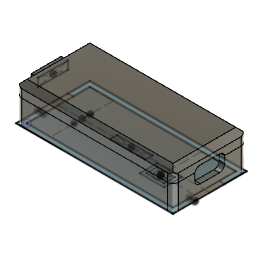
sim_case v2 (Autodesk Fusion 360 design; units mm, degrees)
Autodesk Fusion 360 part; units mm, degrees
sketch "Sketch1" plane through (0, 0, 0) normal (0, 0, 1) x (1, 0, 0)
  line L0 (0, 0) -> (53.5, 0)
  line L1 (53.5, 0) -> (53.5, 23)
  line L2 (53.5, 23) -> (0, 23)
  line L3 (0, 23) -> (0, 0)
  line L4 (-2, -2) -> (55.5, -2)
  line L5 (55.5, -2) -> (55.5, 25)
  line L6 (55.5, 25) -> (-2, 25)
  line L7 (-2, 25) -> (-2, -2)
  line L8 (55.5, 11.5) -> (-2, 11.5) construction
  line L9 (55.5, 11.5) -> (55.5, 17) construction
  line L10 (55.5, 17) -> (53.5, 17)
  line L11 (-2, 11.5) -> (-2, 17) construction
  line L12 (-2, 17) -> (0, 17)
  line L13 (-2, 6) -> (0, 6)
  line L14 (55.5, 6) -> (53.5, 6)
  line L15 (53.5, 23) -> (41, 23) construction
  line L16 (41, 23) -> (41, 8) construction
  line L17 (41, 8) -> (53.5, 8) construction
  line L18 (53.5, 8) -> (53.5, 23) construction
  line L19 (0, 23) -> (8.7, 23) construction
  line L20 (8.7, 23) -> (8.7, 0) construction
  line L21 (8.7, 11.5) -> (8.7, 14.5) construction
  circle A0 centre (8.7, 14.5) radius 0.5
  circle A1 centre (8.7, 8.5) radius 0.5
  circle A2 centre (41, 8) radius 2
  line L22 (33.25, 12.75) -> (20.25, 12.75)
  line L23 (20.25, 12.75) -> (20.25, 10.25)
  line L24 (20.25, 10.25) -> (33.25, 10.25)
  line L25 (33.25, 10.25) -> (33.25, 12.75)
  line L26 (33.25, 12.75) -> (20.25, 10.25) construction
  line L27 (20.25, 12.75) -> (33.25, 10.25) construction
  line L28 (-1, -1) -> (54.5, -1)
  line L29 (54.5, 24) -> (-1, 24)
  line L30 (-1, 17) -> (-1, 6) construction
  line L31 (54.5, -1) -> (54.5, 6)
  line L32 (54.5, 11.5) -> (54.5, 17) construction
  line L33 (54.5, 6) -> (54.5, 11.5) construction
  line L34 (-1, 6) -> (-1, -1)
  line L35 (-1, 24) -> (-1, 17)
  line L36 (54.5, 17) -> (54.5, 24)
  point P0 (41, 8)
  point P1 (8.7, 11.5)
  point P2 (26.75, 11.5)
  dimension "d1" = 53.5
  dimension "d2" = 23
  dimension "d3" = 2
  dimension "d4" = 5.5
  dimension "d5" = 5.5
  dimension "d6" = 12.5
  dimension "d7" = 15
  dimension "d10" = 8.7
  dimension "d11" = 3
  dimension "d12" = 1
  dimension "d13" = 4
  dimension "d14" = 13
  dimension "d15" = 2.5
  constraint horizontal L0
  constraint vertical L1
  constraint horizontal L2
  constraint vertical L3
  constraint coincident L0.start L3.end
  constraint midpoint L5 L8.start
  constraint midpoint L7 L8.end
  constraint perpendicular L8 L9
  constraint coincident L1 L10.end
  constraint perpendicular L1 L10
  constraint perpendicular L8 L11
  constraint coincident L3 L12.end
  constraint perpendicular L3 L12
  constraint symmetric L8 L9.end L14.start
  constraint symmetric L8 L10.end L14.end
  constraint symmetric L8 L11.end L13.start
  constraint symmetric L8 L12.end L13.end
  constraint horizontal L15
  constraint vertical L16
  constraint horizontal L17
  constraint vertical L18
  constraint coincident P0 L16.end
  constraint perpendicular L3 L19
  constraint coincident L0 L20.end
  constraint perpendicular L0 L20
  constraint midpoint L20 P1
  constraint coincident P1 L21.start
  constraint perpendicular L8 L21
  constraint coincident L21.end A0.centre
  constraint symmetric L8 A0 A1
  constraint horizontal L22
  constraint perpendicular L22 L23
  constraint parallel L22 L24
  constraint parallel L23 L25
  constraint coincident L26 P2
  constraint coincident L27 P2
  constraint midpoint L8 P2
  constraint parallel L0 L28
  constraint parallel L1 L31
  constraint parallel L2 L29
  constraint parallel L3 L30
  constraint coincident L14 L31.end
  constraint coincident L8 L32.start
  constraint coincident L13 L30.end
  constraint parallel L3 L34
  constraint coincident L12 L30.start
  constraint parallel L3 L35
  constraint coincident L10 L32.end
  measures "d1" distance of L0.start L0.end
  measures "d2" distance of L0.start L2.end
  measures "d4" distance of L8.start L9.end
  measures "d5" distance of L8.end L11.end
  measures "d6" distance of L1.end L15.end
  measures "d7" distance of L1.end L17.end
  measures "d10" distance of L2.end L19.end
  measures "d11" distance of P1 L21.end
  measures "d12" diameter of A0
  measures "d13" diameter of A2
  measures "d14" distance of L23.end L24.end
  measures "d15" distance of L22.end L23.end
extrude "Extrude1" add sketch "Sketch1" against normal blind 2 makes body 1
extrude "Extrude2" add sketch "Sketch1" along normal blind 9 contours L0 L1 L3 L13 L14 L28 L31 L34 | L1 L2 L3 L10 L12 L29 L35 L36 | L4 L5 L7 L13 L14 L28 L31 L34 | L5 L6 L7 L10 L12 L29 L35 L36 bodies 1
extrude "Extrude3" add sketch "Sketch1" along normal blind 6 contours L3 L7 L12 L13 bodies 1
extrude "Extrude4" add sketch "Sketch1" along normal blind 4.5 contours L1 L5 L10 L14 bodies 1
extrude "Extrude5" add sketch "Sketch1" along normal blind 2 from surface at 12 separate body contours L0 L1 L2 L3 | L0 L1 L3 L13 L14 L28 L31 L34 | L3 L7 L12 L13 | L1 L5 L10 L14 | L1 L2 L3 L10 L12 L29 L35 L36 | L4 L5 L7 L13 L14 L28 L31 L34 | L5 L6 L7 L10 L12 L29 L35 L36 | A0 | A1 | A2 | L22 L23 L24 L25 makes body 2
copy_body "Body->Comp1" bodies 1 removing the originals makes body 3 in component "Cover_top"
copy_body "Body->Comp2" bodies 2 removing the originals makes body 4 in component "Cover_bottom"
extrude "Extrude6" add sketch "Sketch1" along normal up to surface (3 mm away) from surface at 9 separate body contours L0 L1 L3 L13 L14 L28 L31 L34 | L1 L2 L3 L10 L12 L29 L35 L36 | L4 L5 L7 L13 L14 L28 L31 L34 | L5 L6 L7 L10 L12 L29 L35 L36 makes body 5 at (17.1667, -2, 10) makes body 6 at (36.3333, 25, 10)
extrude "Extrude7" add sketch "Sketch1" against normal blind 1.5 from surface at 12 contours L1 L5 L10 L14 bodies 6 5
combine "Combine1" operation add target body 4 tool bodies 6 in component "Cover_bottom"
extrude "Extrude1'" add sketch "Sketch1" against normal blind 3 from surface at 12 contours L3 L7 L12 L13 bodies 4 in component "Cover_bottom"
fillet "Fillet1" radius 2 2 edges at (54.5, 17, 4.5) (54.5, 6, 4.5) on bodies 3 in component "Cover_top"
fillet "Fillet1'" radius 2 2 edges at (54.5, 17, 10.5) (54.5, 6, 10.5) on bodies 4 in component "Cover_bottom"
chamfer "Chamfer1" distance 2 angle 45 4 edges at (26.75, -2, -2) (-2, 11.5, -2) (55.5, 11.5, -2) (26.75, 25, -2) on bodies 3 in component "Cover_top"
chamfer "Chamfer1'" distance 2 angle 45 4 edges at (26.75, -2, 14) (-2, 11.5, 14) (26.75, 25, 14) (55.5, 11.5, 14) on bodies 4 in component "Cover_bottom"
fillet "Fillet2" radius 2 4 edges at (-2, -2, 4.5) (-2, 25, 4.5) (55.5, 25, 4.5) (55.5, -2, 4.5) on bodies 3 in component "Cover_top"
fillet "Fillet2'" radius 2 4 edges at (-2, -2, 10.5) (-2, 25, 10.5) (55.5, 25, 10.5) (55.5, -2, 10.5) on bodies 4 in component "Cover_bottom"
extrude "Extrude1''" add sketch "Sketch1" along normal blind 1 from surface at 9 separate body contours L0 L1 L3 L13 L14 L28 L31 L34 | L1 L2 L3 L10 L12 L29 L35 L36 makes body 7 at (17.8333, 23.6667, 9) makes body 8 at (17.8333, -0.6667, 9) in component "Cover_top"
combine "Combine2" operation cut target body 4 tool bodies 7 8 keep tools in component "Cover_bottom"
combine "Combine1'" operation add target body 3 tool bodies 7 8 in component "Cover_top"
fillet "Fillet3" radius 1 4 edges at (-1, 24, 9.5) (54.5, 24, 9.5) (54.5, -1, 9.5) (-1, -1, 9.5) on bodies 3 in component "Cover_top"
sketch "Sketch2" plane through (0, 0, 0) normal (0, 0, 1) x (-1, 0, 0)
  line L0 (-53.5, 0) -> (-53.5, -23)
  line L1 (-53.5, -23) -> (0, -23)
  line L2 (0, -23) -> (0, 0)
  line L3 (0, 0) -> (-53.5, 0)
  circle A0 centre (-8.7, -14.5) radius 0.5
  circle A1 centre (-8.7, -8.5) radius 0.5
  line L4 (-33.25, -12.75) -> (-33.25, -10.25)
  line L5 (-33.25, -10.25) -> (-20.25, -10.25)
  line L6 (-20.25, -10.25) -> (-20.25, -12.75)
  line L7 (-20.25, -12.75) -> (-33.25, -12.75)
  circle A2 centre (-41, -8) radius 2
  line L8 (-44.25, -10) -> (-37.75, -10)
  line L9 (-37.75, -10) -> (-37.75, -6)
  line L10 (-37.75, -6) -> (-44.25, -6)
  line L11 (-44.25, -6) -> (-44.25, -10)
  line L12 (-44.25, -10) -> (-37.75, -6) construction
  line L13 (-37.75, -10) -> (-44.25, -6) construction
  line L14 (-36.55, -4.8) -> (-45.45, -4.8)
  line L15 (-45.45, -4.8) -> (-45.45, -11.2)
  line L16 (-45.45, -11.2) -> (-36.55, -11.2)
  line L17 (-36.55, -11.2) -> (-36.55, -4.8)
  point P0 (-41, -8)
  dimension "d49" = 6.5
  dimension "d50" = 4
  dimension "d51" = 1.2
  constraint horizontal L8
  constraint perpendicular L8 L9
  constraint parallel L8 L10
  constraint parallel L9 L11
  constraint coincident L12 P0
  constraint coincident L13 P0
  constraint coincident P0 A2.centre
  measures "d49" distance of L9.end L10.end
  measures "d50" distance of L8.end L9.end
extrude "Extrude1'''" add sketch "Sketch2" along normal blind 4.5 and the other way blind 3 separate body contours A2 makes body 9 in component "Button"
extrude "Extrude2'" add sketch "Sketch2" against normal blind 2 from surface at 4.5 contours A2 L8 L9 L10 | A2 L8 L10 L11 | L14 L15 L16 L17 bodies 9 in component "Button"
extrude "Extrude3'" add sketch "Sketch2" along normal blind 4 from surface at 4.5 contours L14 L15 L16 L17 bodies 9 in component "Button"
move_face "OffsetFaces1" offset -0.2 1 faces at (39.0025, 8.0997, 0.6667) on bodies 9 in component "Button"
sketch "Sketch3" plane through (-2, 0, 0) normal (-1, 0, 0) x (0, -1, 0)
  line L0 (-23, 12) -> (-23, 9)
  line L1 (-23, 9) -> (0, 9)
  line L2 (0, 9) -> (0, 12)
  line L3 (0, 12) -> (-23, 12)
  line L4 (-6, 10.5) -> (-17, 10.5)
  line L5 (-17, 10.5) -> (-17, 7.5)
  line L6 (-17, 7.5) -> (-6, 7.5)
  line L7 (-6, 7.5) -> (-6, 10.5)
  line L8 (-6, 10.5) -> (-17, 7.5) construction
  line L9 (-17, 10.5) -> (-6, 7.5) construction
  point P0 (-11.5, 9)
  dimension "d63" = 11
  dimension "d64" = 3
  constraint horizontal L4
  constraint perpendicular L4 L5
  constraint parallel L4 L6
  constraint parallel L5 L7
  constraint coincident L8 P0
  constraint coincident L9 P0
  constraint midpoint L1 P0
  measures "d63" distance of L5.end L6.end
  measures "d64" distance of L4.end L5.end
extrude "Extrude2''" add sketch "Sketch3" along normal blind 2.5 contours L1 L4 L5 L7 bodies 4 in component "Cover_bottom"
extrude "Extrude4'" cut 1 faces at (42.4833, 11.2, 4.5) along direction (0, -1, 0) blind 0.4 on bodies 9 bodies 9 in component "Button"
component "Cover_top" placed x (1, 0, 0) y (0, 1, 0) z (0, 0, 1) at (0, 0, 0)
component "Cover_bottom" placed x (1, 0, 0) y (0, 1, 0) z (0, 0, 1) at (0, 0, 0)
component "Button" placed x (1, 0, 0) y (0, 1, 0) z (0, 0, 1) at (0, 0, 0)
